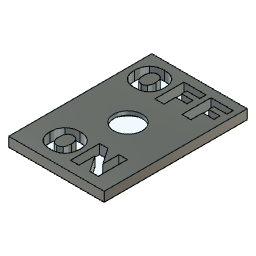
OFFONPLATE (Autodesk Fusion 360 design; units mm, degrees)
Autodesk Fusion 360 part; units mm, degrees
sketch "Sketch1" plane through (0, 0, 0) normal (0, 0, 1) x (1, 0, 0)
  line L0 (0, 0) -> (20, 0)
  line L1 (20, 0) -> (20, 30)
  line L2 (20, 30) -> (0, 30)
  line L3 (0, 30) -> (0, 0)
  dimension "d1" = 30
  dimension "d2" = 20
  constraint horizontal L0
  constraint vertical L1
  constraint horizontal L2
  constraint vertical L3
  constraint coincident L0.start L3.end
  measures "d1" distance of L0.start L2.end
  measures "d2" distance of L1.end L2.end
extrude "Extrude1" add sketch "Sketch1" along normal blind 2 makes body 1
sketch "Sketch2" plane through (0, 0, 2) normal (0, 0, 1) x (-1, 0, 0)
  line L0 (0, -30) -> (0, 0)
  line L1 (0, 0) -> (-20, 0)
  line L2 (-20, 0) -> (-20, -30)
  line L3 (-20, -30) -> (0, -30)
  circle A0 centre (-10, -15) radius 3
  dimension "d5" = 6
  dimension "d6" = 15
  dimension "d7" = 10
  measures "d5" diameter of A0
  measures "d6" distance of L1 A0.centre
  measures "d7" distance of L2 A0.centre
extrude "Extrude2" cut sketch "Sketch2" against normal blind 2 contours A0 bodies 1
sketch "Sketch3" plane through (0, 0, 2) normal (0, 0, 1) x (-1, 0, 0)
  circle A0 centre (-10, -15) radius 3
  line L0 (0, -30) -> (0, 0)
  line L1 (0, 0) -> (-20, 0)
  line L2 (-20, 0) -> (-20, -30)
  line L3 (-20, -30) -> (0, -30)
sketch "Sketch4" plane through (0, 0, 2) normal (0, 0, 1) x (-1, 0, 0)
  line L0 (-1.2, -22) -> (-18.63, -22) construction
  line L1 (-18.63, -22) -> (-18.63, -30.5) construction
  line L2 (-18.63, -30.5) -> (-1.2, -30.5) construction
  line L3 (-1.2, -30.5) -> (-1.2, -22) construction
  line L4 (0, -30) -> (0, 0)
  line L5 (-3.5, -2) -> (-14.1484, -2) construction
  line L6 (-14.1484, -2) -> (-14.1484, -10.5) construction
  line L7 (-14.1484, -10.5) -> (-3.5, -10.5) construction
  line L8 (-3.5, -10.5) -> (-3.5, -2) construction
  point P0 (-10, -15)
  dimension "d11" = 1.2
  dimension "d12" = 3.5
  dimension "d13" = 4.5
  dimension "d14" = 7
  text T0 "OFF" font "Arial Black" height 8.5 align ink ink in box 0 x 0 at (-1.2, -22) x (-1, 0) y (0, -1) spacing 1 height is em
  text T1 "ON" font "Arial Black" height 8.5 align ink ink in box 0 x 0 at (-3.5, -2) x (-1, 0) y (0, -1) spacing 1 height is em
  constraint perpendicular L0 L1
  constraint parallel L0 L2
  constraint parallel L1 L3
  constraint perpendicular L5 L6
  constraint parallel L5 L7
  constraint parallel L6 L8
  measures "d11" distance of L3 L4
  measures "d12" distance of L4 L8
  measures "d13" distance of L7 P0
  measures "d14" distance of L0 P0
extrude "Extrude3" cut sketch "Sketch4" against normal blind 2 text T1 T0 bodies 1 makes body 2 at (4.3266, 23.9034, 0) makes body 3 at (6.6266, 3.9034, 0)
sketch "Sketch5" plane through (0, 0, 0) normal (0, 0, -1) x (1, 0, 0)
  line L0 (14.2049, -22.1138) -> (16.0933, -22.1138)
  line L1 (16.0933, -22.1138) -> (16.0933, -24.5998)
  line L2 (16.0933, -24.5998) -> (18.4507, -24.5998)
  line L3 (18.4507, -24.5998) -> (18.4507, -25.8284)
  line L4 (18.4507, -25.8284) -> (16.0933, -25.8284)
  line L5 (16.0933, -25.8284) -> (16.0933, -26.8909)
  line L6 (16.0933, -26.8909) -> (18.8533, -26.8909)
  line L7 (18.8533, -26.8909) -> (18.8533, -28.1982)
  line L8 (18.8533, -28.1982) -> (14.2049, -28.1982)
  line L9 (14.2049, -28.1982) -> (14.2049, -22.1138)
  line L10 (10.8396, -2.1138) -> (12.6077, -2.1138)
  line L11 (12.6077, -2.1138) -> (12.6077, -5.4546)
  line L12 (12.6077, -5.4546) -> (14.8862, -2.1138)
  line L13 (14.8862, -2.1138) -> (16.6584, -2.1138)
  line L14 (16.6584, -2.1138) -> (16.6584, -8.1982)
  line L15 (16.6584, -8.1982) -> (14.8862, -8.1982)
  line L16 (14.8862, -8.1982) -> (14.8862, -4.832)
  line L17 (14.8862, -4.832) -> (12.5952, -8.1982)
  line L18 (12.5952, -8.1982) -> (10.8396, -8.1982)
  line L19 (10.8396, -8.1982) -> (10.8396, -2.1138)
  spline S0 degree 3 poles (3.9292, -3.3755) (4.0766, -3.1563) (4.3642, -2.7287) (4.807, -2.4659) (5.0228, -2.3379) knots -0.152443 -0.152443 -0.152443 -0.152443 -0.074302 0 0 0 0
  spline S1 degree 3 poles (5.0228, -2.3379) (5.2745, -2.2424) (5.8225, -2.0345) (6.4092, -2.0186) (6.7266, -2.01) knots -0.174594 -0.174594 -0.174594 -0.174594 -0.094415 0 0 0 0
  spline S2 degree 3 poles (6.7266, -2.01) (7.0411, -2.021) (7.6297, -2.0415) (8.1675, -2.2791) (8.4178, -2.3898) knots -0.174761 -0.174761 -0.174761 -0.174761 -0.08136 0 0 0 0
  spline S3 degree 3 poles (8.4178, -2.3898) (8.6306, -2.5287) (9.0552, -2.8061) (9.3222, -3.2372) (9.4554, -3.4523) knots -0.150133 -0.150133 -0.150133 -0.150133 -0.074905 0 0 0 0
  spline S4 degree 3 poles (9.4554, -3.4523) (9.56, -3.7086) (9.7881, -4.2684) (9.8052, -4.8736) (9.8144, -5.2017) knots -0.179877 -0.179877 -0.179877 -0.179877 -0.097481 0 0 0 0
  spline S5 degree 3 poles (9.8144, -5.2017) (9.7903, -5.6536) (9.745, -6.501) (9.2321, -7.1729) (8.9927, -7.4864) knots -0.247871 -0.247871 -0.247871 -0.247871 -0.115683 0 0 0 0
  spline S6 degree 3 poles (8.9927, -7.4864) (8.6729, -7.7239) (7.9812, -8.2378) (7.1167, -8.2795) (6.6518, -8.302) knots -0.2529 -0.2529 -0.2529 -0.2529 -0.13601 0 0 0 0
  spline S7 degree 3 poles (6.6518, -8.302) (6.1956, -8.2773) (5.3388, -8.231) (4.6582, -7.7137) (4.3401, -7.4719) knots -0.250702 -0.250702 -0.250702 -0.250702 -0.1172 0 0 0 0
  spline S8 degree 3 poles (4.3401, -7.4719) (4.0983, -7.153) (3.5801, -6.4698) (3.5344, -5.6102) (3.51, -5.1518) knots -0.251493 -0.251493 -0.251493 -0.251493 -0.134116 0 0 0 0
  spline S9 degree 3 poles (3.51, -5.1518) (3.5222, -4.8205) (3.5451, -4.1997) (3.8071, -3.6375) (3.9292, -3.3755) knots -0.18416 -0.18416 -0.18416 -0.18416 -0.085858 0 0 0 0
  line L20 (8.5354, -22.1138) -> (10.4239, -22.1138)
  line L21 (10.4239, -22.1138) -> (10.4239, -24.5998)
  line L22 (10.4239, -24.5998) -> (12.7813, -24.5998)
  line L23 (12.7813, -24.5998) -> (12.7813, -25.8284)
  line L24 (12.7813, -25.8284) -> (10.4239, -25.8284)
  line L25 (10.4239, -25.8284) -> (10.4239, -26.8909)
  line L26 (10.4239, -26.8909) -> (13.1839, -26.8909)
  line L27 (13.1839, -26.8909) -> (13.1839, -28.1982)
  line L28 (13.1839, -28.1982) -> (8.5354, -28.1982)
  line L29 (8.5354, -28.1982) -> (8.5354, -22.1138)
  spline S10 degree 3 poles (1.6292, -23.3755) (1.7766, -23.1563) (2.0642, -22.7287) (2.507, -22.4659) (2.7228, -22.3379) knots -0.152443 -0.152443 -0.152443 -0.152443 -0.074302 0 0 0 0
  spline S11 degree 3 poles (2.7228, -22.3379) (2.9745, -22.2424) (3.5225, -22.0345) (4.1092, -22.0186) (4.4266, -22.01) knots -0.174594 -0.174594 -0.174594 -0.174594 -0.094415 0 0 0 0
  spline S12 degree 3 poles (4.4266, -22.01) (4.7411, -22.021) (5.3297, -22.0415) (5.8675, -22.2791) (6.1178, -22.3898) knots -0.174761 -0.174761 -0.174761 -0.174761 -0.08136 0 0 0 0
  spline S13 degree 3 poles (6.1178, -22.3898) (6.3306, -22.5287) (6.7552, -22.8061) (7.0222, -23.2372) (7.1554, -23.4523) knots -0.150133 -0.150133 -0.150133 -0.150133 -0.074905 0 0 0 0
  spline S14 degree 3 poles (7.1554, -23.4523) (7.26, -23.7086) (7.4881, -24.2684) (7.5052, -24.8736) (7.5144, -25.2017) knots -0.179877 -0.179877 -0.179877 -0.179877 -0.097481 0 0 0 0
  spline S15 degree 3 poles (7.5144, -25.2017) (7.4903, -25.6536) (7.445, -26.501) (6.9321, -27.1729) (6.6927, -27.4864) knots -0.247871 -0.247871 -0.247871 -0.247871 -0.115683 0 0 0 0
  spline S16 degree 3 poles (6.6927, -27.4864) (6.3729, -27.7239) (5.6812, -28.2378) (4.8167, -28.2795) (4.3518, -28.302) knots -0.2529 -0.2529 -0.2529 -0.2529 -0.13601 0 0 0 0
  spline S17 degree 3 poles (4.3518, -28.302) (3.8956, -28.2773) (3.0388, -28.231) (2.3582, -27.7137) (2.0401, -27.4719) knots -0.250702 -0.250702 -0.250702 -0.250702 -0.1172 0 0 0 0
  spline S18 degree 3 poles (2.0401, -27.4719) (1.7983, -27.153) (1.2801, -26.4698) (1.2344, -25.6102) (1.21, -25.1518) knots -0.251493 -0.251493 -0.251493 -0.251493 -0.134116 0 0 0 0
  spline S19 degree 3 poles (1.21, -25.1518) (1.2222, -24.8205) (1.2451, -24.1997) (1.5071, -23.6375) (1.6292, -23.3755) knots -0.18416 -0.18416 -0.18416 -0.18416 -0.085858 0 0 0 0
  circle A0 centre (10, -15) radius 3
  line L30 (0, 0) -> (0, -30)
  line L31 (0, -30) -> (20, -30)
  line L32 (20, -30) -> (20, 0)
  line L33 (20, 0) -> (0, 0)
  circle A1 centre (10, -15) radius 4.5
  dimension "d17" = 9
  constraint concentric A0 A1
  measures "d17" diameter of A1
extrude "Extrude4" cut sketch "Sketch5" against normal blind 1.2 contours A1 bodies 1
